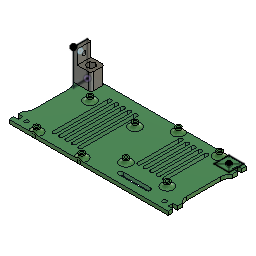
Support_RPI (Autodesk Fusion 360 design; units mm, degrees)
Autodesk Fusion 360 part; units mm, degrees
note: some values were not read from the file. Chosen so that the rebuilt part matches the saved one: that a step has no effect. Set by a fixed rule: which sketch regions a step uses.
sketch "Sketch1" plane through (0, 0, 0) normal (0, 0, 1) x (1, 0, 0) in component "Support_RPI"
  line L0 (-82.5, 42.5) -> (82.5, 42.5)
  line L1 (82.5, 42.5) -> (82.5, -42.5)
  line L2 (82.5, -42.5) -> (-82.5, -42.5)
  line L3 (-82.5, -42.5) -> (-82.5, 42.5)
  line L4 (-82.5, 42.5) -> (82.5, -42.5) construction
  line L5 (82.5, 42.5) -> (-82.5, -42.5) construction
  line L6 (0, 42.5) -> (0, -42.5) construction
  line L7 (-82.5, 42.5) -> (-86.5, 42.5)
  line L8 (-86.5, 42.5) -> (-86.5, 27.5)
  line L9 (-86.5, 27.5) -> (-82.5, 27.5)
  line L10 (-82.5, 27.5) -> (-82.5, 42.5)
  line L11 (-82.5, -42.5) -> (-86.5, -42.5)
  line L12 (-86.5, -42.5) -> (-86.5, -27.5)
  line L13 (-86.5, -27.5) -> (-82.5, -27.5)
  line L14 (-82.5, -27.5) -> (-82.5, -42.5)
  line L15 (82.5, 42.5) -> (86.5, 42.5)
  line L16 (86.5, 42.5) -> (86.5, 27.5)
  line L17 (86.5, 27.5) -> (82.5, 27.5)
  line L18 (82.5, 27.5) -> (82.5, 42.5)
  line L19 (82.5, -42.5) -> (86.5, -42.5)
  line L20 (86.5, -27.5) -> (82.5, -27.5)
  line L21 (82.5, -27.5) -> (82.5, -42.5)
  line L22 (86.5, -42.5) -> (86.5, -27.5)
  line L23 (-82.5, -42.5) -> (-67.5, -42.5)
  line L24 (-67.5, -42.5) -> (-67.5, -27.5)
  line L25 (-67.5, -27.5) -> (-82.5, -27.5)
  line L26 (-82.5, -27.5) -> (-82.5, -42.5)
  line L27 (-82.5, 42.5) -> (-67.5, 42.5)
  line L28 (-67.5, 42.5) -> (-67.5, 27.5)
  line L29 (-67.5, 27.5) -> (-82.5, 27.5)
  line L30 (-82.5, 27.5) -> (-82.5, 42.5)
  line L31 (82.5, 42.5) -> (67.5, 42.5)
  line L32 (67.5, 42.5) -> (67.5, 27.5)
  line L33 (67.5, 27.5) -> (82.5, 27.5)
  line L34 (82.5, 27.5) -> (82.5, 42.5)
  line L35 (82.5, -42.5) -> (67.5, -42.5)
  line L36 (67.5, -27.5) -> (82.5, -27.5)
  line L37 (82.5, -27.5) -> (82.5, -42.5)
  line L38 (67.5, -42.5) -> (67.5, -27.5)
  line L39 (-82.5, 27.5) -> (-67.5, 42.5) construction
  line L40 (-82.5, -42.5) -> (-67.5, -27.5) construction
  circle A0 centre (-75, 35) radius 2.1
  circle A1 centre (-75, -35) radius 2.1
  circle A2 centre (75, 35) radius 2.1
  circle A3 centre (75, -35) radius 2.1
  line L41 (-82.5, 42.5) -> (-86.5, 27.5) construction
  line L42 (-81.5, 32.5) -> (-87.5, 32.5)
  line L43 (-87.5, 32.5) -> (-87.5, 37.5)
  line L44 (-87.5, 37.5) -> (-81.5, 37.5)
  line L45 (-81.5, 37.5) -> (-81.5, 32.5)
  line L46 (-81.5, 32.5) -> (-87.5, 37.5) construction
  line L47 (-87.5, 32.5) -> (-81.5, 37.5) construction
  line L48 (-82.5, -27.5) -> (-86.5, -42.5) construction
  line L49 (-81.5, -37.5) -> (-87.5, -37.5)
  line L50 (-87.5, -37.5) -> (-87.5, -32.5)
  line L51 (-87.5, -32.5) -> (-81.5, -32.5)
  line L52 (-81.5, -32.5) -> (-81.5, -37.5)
  line L53 (-81.5, -37.5) -> (-87.5, -32.5) construction
  line L54 (-87.5, -37.5) -> (-81.5, -32.5) construction
  line L55 (81.5, -37.5) -> (87.5, -37.5)
  line L56 (87.5, -37.5) -> (87.5, -32.5)
  line L57 (87.5, -32.5) -> (81.5, -32.5)
  line L58 (81.5, -32.5) -> (81.5, -37.5)
  line L59 (87.5, 37.5) -> (81.5, 37.5)
  line L60 (81.5, 37.5) -> (81.5, 32.5)
  line L61 (87.5, 32.5) -> (87.5, 37.5)
  line L62 (81.5, 32.5) -> (87.5, 32.5)
  point P0 (-82.5, 35)
  point P1 (-84.5, 35)
  point P2 (-84.5, -35)
  dimension "d1" = 85
  dimension "d2" = 165
  dimension "d167" = 15
  dimension "d168" = 4
  dimension "d169" = 15
  dimension "d170" = 4
  dimension "d187" = 15
  dimension "d188" = 15
  dimension "d189" = 15
  dimension "d190" = 15
  dimension "d201" = 4.2
  dimension "d202" = 4.2
  dimension "d206" = 6
  dimension "d207" = 5
  dimension "d208" = 6
  dimension "d209" = 5
  constraint perpendicular L0 L1
  constraint parallel L1 L3
  constraint horizontal L0
  constraint midpoint L2 L6.end
  constraint midpoint origin L5
  constraint midpoint origin L4
  constraint midpoint origin L6
  constraint horizontal L7
  constraint vertical L8
  constraint horizontal L9
  constraint vertical L10
  constraint horizontal L11
  constraint vertical L12
  constraint horizontal L13
  constraint vertical L14
  constraint symmetric L0.start L6 L0.end
  constraint symmetric L2.end L6 L1.end
  constraint symmetric L6 L7.end L15.end
  constraint symmetric L6 L8.end L16.end
  constraint symmetric L6 L9.end L17.end
  constraint symmetric L6 L11.end L19.end
  constraint symmetric L6 L12.end L20.start
  constraint symmetric L6 L13.end L20.end
  constraint horizontal L23
  constraint vertical L24
  constraint horizontal L25
  constraint vertical L26
  constraint horizontal L27
  constraint vertical L28
  constraint horizontal L29
  constraint vertical L30
  constraint symmetric L6 L23.end L35.end
  constraint symmetric L6 L24.end L36.start
  constraint symmetric L6 L27.end L31.end
  constraint symmetric L6 L28.end L32.end
  constraint midpoint L39 A0.centre
  constraint midpoint L40 A1.centre
  constraint symmetric L6 A0 A2
  constraint symmetric L6 A1 A3
  constraint midpoint L10 P0
  constraint horizontal L42
  constraint perpendicular L42 L43
  constraint parallel L42 L44
  constraint parallel L43 L45
  constraint coincident L46 P1
  constraint coincident L47 P1
  constraint midpoint L41 P1
  constraint horizontal L49
  constraint perpendicular L49 L50
  constraint parallel L49 L51
  constraint parallel L50 L52
  constraint coincident L53 P2
  constraint coincident L54 P2
  constraint midpoint L48 P2
  constraint symmetric L6 L42.start L60.end
  constraint symmetric L6 L42.end L61.start
  constraint symmetric L6 L43.end L59.start
  constraint symmetric L6 L44.end L59.end
  constraint symmetric L6 L49.start L55.start
  constraint symmetric L6 L49.end L55.end
  constraint symmetric L6 L50.end L56.end
  constraint symmetric L6 L51.end L57.end
  measures "d1" distance of L0.end L1.end
  measures "d2" distance of L1.end L2.end
  measures "d121" distance of L0.end
  measures "d122" distance of L0.end
  measures "d128" diameter of L0.end
  measures "d167" distance of L7.end L8.end
  measures "d168" distance of L0.start L7.end
  measures "d169" distance of L11.end L12.end
  measures "d170" distance of L2.end L11.end
  measures "d187" distance of L2.end L23.end
  measures "d188" distance of L2.end L13.end
  measures "d189" distance of L0.start L27.end
  measures "d190" distance of L0.start L9.end
  measures "d201" diameter of A0
  measures "d202" diameter of A1
  measures "d206" distance of L43.end L44.end
  measures "d207" distance of L42.end L43.end
  measures "d208" distance of L50.end L51.end
  measures "d209" distance of L49.end L50.end
  measures "d210" distance of L0.end
extrude "Extrude1" add sketch "Sketch1" along normal blind 4 contours L0 L3 L10 L27 L28 L29 L30 L42 L44 L45 | L3 L7 L8 L10 L30 L44 | L0 L1 L2 L3 L24 L25 L28 L29 L32 L33 L36 L38 | L0 L1 L18 L31 L32 L33 L34 L59 L60 L62 | L3 L8 L9 L10 L30 L42 | L1 L15 L16 L18 L34 L59 | L1 L16 L17 L18 L34 L62 | L2 L3 L14 L23 L24 L25 L26 L49 L51 L52 | L3 L12 L13 L14 L26 L51 | L1 L20 L21 L22 L37 L57 | L1 L2 L21 L35 L36 L37 L38 L55 L57 L58 | L3 L11 L12 L14 L26 L49 | L1 L19 L21 L22 L37 L55 makes body 1 in component "Support_RPI"
sketch "Sketch2" plane through (0, 0, 4) normal (0, 0, 1) x (-1, 0, 0) in component "Support_RPI"
  line L0 (86.5, 42.5) -> (-86.5, 42.5)
  line L1 (-82.5, 27.5) -> (-82.5, -27.5)
  line L2 (-86.5, -42.5) -> (86.5, -42.5)
  circle A0 centre (11, -19) radius 3
  circle A1 centre (11, -19) radius 1.6
  circle A2 centre (60, -19) radius 1.6
  circle A3 centre (60, 39) radius 1.6
  circle A4 centre (60, 39) radius 3
  circle A5 centre (11, 39) radius 1.6
  circle A6 centre (11, 39) radius 3
  line L3 (60, -19) -> (11, -19) construction
  line L4 (11, -19) -> (11, 39) construction
  line L5 (11, 39) -> (60, 39) construction
  line L6 (60, 39) -> (60, -19) construction
  line L7 (60, 10) -> (11, 10) construction
  line L8 (37.5, -30) -> (37.5, 30)
  arc A7 (37.5, 30) -> (33.5, 30) centre (35.5, 30) ccw
  line L9 (33.5, 30) -> (33.5, -30)
  arc A8 (33.5, -30) -> (37.5, -30) centre (35.5, -30) ccw
  line L10 (35.5, -30) -> (35.5, 30) construction
  line L11 (23.5, -30) -> (23.5, 30)
  arc A9 (23.5, 30) -> (19.5, 30) centre (21.5, 30) ccw
  line L12 (19.5, 30) -> (19.5, -30)
  arc A10 (19.5, -30) -> (23.5, -30) centre (21.5, -30) ccw
  line L13 (30.5, -30) -> (30.5, 30)
  arc A11 (30.5, 30) -> (26.5, 30) centre (28.5, 30) ccw
  line L14 (26.5, 30) -> (26.5, -30)
  arc A12 (26.5, -30) -> (30.5, -30) centre (28.5, -30) ccw
  line L15 (44.5, -30) -> (44.5, 30)
  arc A13 (44.5, 30) -> (40.5, 30) centre (42.5, 30) ccw
  line L16 (40.5, 30) -> (40.5, -30)
  arc A14 (40.5, -30) -> (44.5, -30) centre (42.5, -30) ccw
  circle A15 centre (60, -19) radius 3
  line L17 (-82.5, -42.5) -> (-82.5, 42.5) construction
  line L18 (5.5, 42.5) -> (65.5, 42.5) construction
  line L19 (65.5, 42.5) -> (65.5, -42.5) construction
  line L20 (65.5, -42.5) -> (5.5, -42.5) construction
  line L21 (5.5, -42.5) -> (5.5, 42.5) construction
  line L22 (5.5, 42.5) -> (65.5, -42.5) construction
  line L23 (65.5, 42.5) -> (5.5, -42.5) construction
  line L24 (0, 0) -> (35.5, 0) construction
  line L25 (-62.5, 19.5) -> (-17.5, 19.5) construction
  line L26 (-17.5, 19.5) -> (-17.5, -37.5) construction
  line L27 (-17.5, -37.5) -> (-62.5, -37.5) construction
  line L28 (-62.5, -37.5) -> (-62.5, 19.5) construction
  line L29 (-62.5, 19.5) -> (-17.5, -37.5) construction
  line L30 (-17.5, 19.5) -> (-62.5, -37.5) construction
  circle A16 centre (-17.5, -37.5) radius 1.6
  circle A17 centre (-62.5, -37.5) radius 1.6
  circle A18 centre (-17.5, 19.5) radius 1.6
  circle A19 centre (-62.5, 19.5) radius 1.6
  circle A20 centre (-17.5, -37.5) radius 3
  circle A21 centre (-62.5, -37.5) radius 3
  circle A22 centre (-17.5, 19.5) radius 3
  circle A23 centre (-62.5, 19.5) radius 3
  line L31 (51.5, -30) -> (51.5, 30)
  arc A24 (51.5, 30) -> (47.5, 30) centre (49.5, 30) ccw
  line L32 (47.5, 30) -> (47.5, -30)
  arc A25 (47.5, -30) -> (51.5, -30) centre (49.5, -30) ccw
  line L33 (-38, -31.5) -> (-38, 13.5)
  arc A26 (-38, 13.5) -> (-42, 13.5) centre (-40, 13.5) ccw
  line L34 (-42, 13.5) -> (-42, -31.5)
  arc A27 (-42, -31.5) -> (-38, -31.5) centre (-40, -31.5) ccw
  line L35 (-40, -31.5) -> (-40, 13.5) construction
  line L36 (-52, -31.5) -> (-52, 13.5)
  arc A28 (-52, 13.5) -> (-56, 13.5) centre (-54, 13.5) ccw
  line L37 (-56, 13.5) -> (-56, -31.5)
  arc A29 (-56, -31.5) -> (-52, -31.5) centre (-54, -31.5) ccw
  line L38 (-45, -31.5) -> (-45, 13.5)
  arc A30 (-45, 13.5) -> (-49, 13.5) centre (-47, 13.5) ccw
  line L39 (-49, 13.5) -> (-49, -31.5)
  arc A31 (-49, -31.5) -> (-45, -31.5) centre (-47, -31.5) ccw
  line L40 (-31, -31.5) -> (-31, 13.5)
  arc A32 (-31, 13.5) -> (-35, 13.5) centre (-33, 13.5) ccw
  line L41 (-35, 13.5) -> (-35, -31.5)
  arc A33 (-35, -31.5) -> (-31, -31.5) centre (-33, -31.5) ccw
  line L42 (-24, -31.5) -> (-24, 13.5)
  arc A34 (-24, 13.5) -> (-28, 13.5) centre (-26, 13.5) ccw
  line L43 (-28, 13.5) -> (-28, -31.5)
  arc A35 (-28, -31.5) -> (-24, -31.5) centre (-26, -31.5) ccw
  line L44 (-25, 35) -> (-55, 35)
  arc A36 (-55, 35) -> (-55, 30) centre (-55, 32.5) ccw
  line L45 (-55, 30) -> (-25, 30)
  arc A37 (-25, 30) -> (-25, 35) centre (-25, 32.5) ccw
  line L46 (-25, 32.5) -> (-55, 32.5) construction
  line L47 (-40, -9) -> (-40, 32.5) construction
  line L48 (-40, 32.5) -> (-40, 42.5) construction
  circle A38 centre (-75, 35) radius 2.1
  circle A39 centre (75, 35) radius 2.1
  circle A40 centre (75, -35) radius 2.1
  circle A41 centre (-75, -35) radius 2.1
  line L49 (-86.5, 42.5) -> (-86.5, 37.5)
  line L50 (-86.5, 27.5) -> (-82.5, 27.5)
  line L51 (-82.5, -27.5) -> (-86.5, -27.5)
  line L52 (-86.5, -27.5) -> (-86.5, -32.5)
  line L53 (86.5, -42.5) -> (86.5, -37.5)
  line L54 (86.5, -27.5) -> (82.5, -27.5)
  line L55 (82.5, 27.5) -> (86.5, 27.5)
  line L56 (86.5, 27.5) -> (86.5, 32.5)
  line L57 (86.5, -37.5) -> (81.5, -37.5)
  line L58 (81.5, -32.5) -> (86.5, -32.5)
  line L59 (86.5, -32.5) -> (86.5, -27.5)
  line L60 (82.5, -27.5) -> (82.5, 27.5)
  line L61 (81.5, -37.5) -> (81.5, -32.5)
  line L62 (86.5, 32.5) -> (81.5, 32.5)
  line L63 (81.5, 32.5) -> (81.5, 37.5)
  line L64 (81.5, 37.5) -> (86.5, 37.5)
  line L65 (86.5, 37.5) -> (86.5, 42.5)
  line L66 (-86.5, 37.5) -> (-81.5, 37.5)
  line L67 (-81.5, 37.5) -> (-81.5, 32.5)
  line L68 (-81.5, 32.5) -> (-86.5, 32.5)
  line L69 (-86.5, 32.5) -> (-86.5, 27.5)
  line L70 (-86.5, -32.5) -> (-81.5, -32.5)
  line L71 (-81.5, -32.5) -> (-81.5, -37.5)
  line L72 (-81.5, -37.5) -> (-86.5, -37.5)
  line L73 (-86.5, -37.5) -> (-86.5, -42.5)
  line L74 (67.5, -42.5) -> (67.5, 42.5) construction
  line L75 (-67.5, -42.5) -> (-67.5, 42.5) construction
  point P0 (35.5, 10)
  point P1 (35.5, 0)
  point P2 (-40, -9)
  point P3 (-40, -9)
  point P4 (-40, 32.5)
  dimension "d5" = 6
  dimension "d6" = 3.2
  dimension "d8" = 3.2
  dimension "d9" = 6
  dimension "d10" = 3.2
  dimension "d11" = 6
  dimension "d12" = 3.2
  dimension "d16" = 49
  dimension "d17" = 58
  dimension "d65" = 4
  dimension "d68" = 7
  dimension "d69" = 0
  dimension "d128" = 6
  dimension "d131" = 3.5
  dimension "d134" = 15
  dimension "d138" = 60
  dimension "d139" = 85
  dimension "d140" = 57
  dimension "d141" = 45
  dimension "d142" = 5
  dimension "d143" = 3.2
  dimension "d144" = 3.2
  dimension "d145" = 3.2
  dimension "d146" = 3.2
  dimension "d147" = 6
  dimension "d148" = 6
  dimension "d149" = 6
  dimension "d150" = 6
  dimension "d151" = 30
  dimension "d152" = 2
  dimension "d153" = 45
  dimension "d156" = 7
  dimension "d157" = 0
  dimension "d162" = 2.5
  dimension "d163" = 10
  dimension "d164" = 30
  dimension "d226" = 15
  dimension "d227" = 15
  dimension "d228" = 2
  dimension "d229" = 5
  constraint concentric A0 A1
  constraint concentric A3 A4
  constraint concentric A5 A6
  constraint horizontal L3
  constraint vertical L4
  constraint horizontal L5
  constraint vertical L6
  constraint coincident A0.centre A1.centre
  constraint coincident A3.centre A4.centre
  constraint coincident A5.centre A6.centre
  constraint midpoint L6 L7.start
  constraint midpoint L4 L7.end
  constraint tangent L8 A7
  constraint tangent A7 L9
  constraint parallel L8 L9
  constraint tangent L9 A8
  constraint tangent L8 A8
  constraint perpendicular L7 L10
  constraint midpoint L7 P0
  constraint concentric A2 A15
  constraint coincident L6 A2.centre
  constraint coincident A2.centre L3.start
  constraint coincident L2 L17.start
  constraint coincident L0 L17.end
  constraint perpendicular L0 L17
  constraint horizontal L18
  constraint perpendicular L18 L19
  constraint parallel L18 L20
  constraint parallel L19 L21
  constraint coincident L22 P1
  constraint coincident L23 P1
  constraint coincident L10 P1
  constraint coincident L24.start origin
  constraint coincident P1 L24.end
  constraint horizontal L24
  constraint horizontal L25
  constraint perpendicular L25 L26
  constraint parallel L25 L27
  constraint parallel L26 L28
  constraint coincident L29 P3
  constraint coincident L30 P3
  constraint coincident L26.end L27.start
  constraint coincident L27.end L28.start
  constraint coincident L25.end L26.start
  constraint coincident L25.start L28.end
  constraint concentric A16 A20
  constraint concentric A17 A21
  constraint concentric A18 A22
  constraint concentric A19 A23
  constraint coincident L10 P0
  constraint midpoint L10 P1
  constraint tangent L33 A26
  constraint tangent A26 L34
  constraint parallel L33 L34
  constraint tangent L34 A27
  constraint tangent L33 A27
  constraint coincident P3 P2
  constraint midpoint L35 P3
  constraint tangent L44 A36
  constraint tangent A36 L45
  constraint parallel L44 L45
  constraint tangent L45 A37
  constraint tangent L44 A37
  constraint perpendicular L43 L46
  constraint midpoint L46 P4
  constraint coincident P4 L47.end
  constraint vertical L47
  constraint coincident L0 L48.end
  constraint perpendicular L0 L48
  constraint vertical L35
  constraint coincident L2 L74.start
  constraint coincident L0 L74.end
  constraint perpendicular L0 L74
  constraint coincident L2 L75.start
  constraint coincident L0 L75.end
  constraint perpendicular L0 L75
  constraint coincident L1.end L17
  measures "d5" diameter of A0
  measures "d6" diameter of A1
  measures "d8" diameter of A2
  measures "d9" diameter of A4
  measures "d10" diameter of A3
  measures "d11" diameter of A6
  measures "d12" diameter of A5
  measures "d16" distance of A2.centre A0.centre
  measures "d17" distance of A2.centre A3.centre
  measures "d65" diameter of A7
  measures "d128" diameter of A15
  measures "d131" distance of L0 L5
  measures "d134" distance of L1.end L17.start
  measures "d138" distance of L18.start L18.end
  measures "d139" distance of L18.start L20.end
  measures "d140" distance of L25.start L27.end
  measures "d141" distance of L26.end L27.end
  measures "d142" distance of L2 L27.end
  measures "d143" diameter of A16
  measures "d144" diameter of A17
  measures "d145" diameter of A18
  measures "d146" diameter of A19
  measures "d147" diameter of A20
  measures "d148" diameter of A21
  measures "d149" diameter of A22
  measures "d150" diameter of A23
  measures "d151" distance of A8.centre P1
  measures "d152" radius of A27
  measures "d153" distance of A27.centre A26.centre
  measures "d162" radius of A36
  measures "d163" distance of P4 L48.end
  measures "d164" distance of A37.centre A36.centre
  measures "d226" horizontal distance of L54.end L74.start
  measures "d227" distance of L17.start L75.start
  measures "d228" distance of L19.end L74.start
  measures "d229" horizontal distance of L27.end L75.start
extrude "Extrude2" add sketch "Sketch2" along normal blind 5 contours A0 | A4 | A6 | A15 | A20 | A21 | A22 | A23 bodies 1 in component "Support_RPI"
extrude "Extrude8" cut sketch "Sketch2" against normal through all contours L8 A7 L9 A8 | L11 A9 L12 A10 | L13 A11 L14 A12 | L15 A13 L16 A14 | L31 A24 L32 A25 | L33 A26 L34 A27 | L36 A28 L37 A29 | L38 A30 L39 A31 | L40 A32 L41 A33 | L42 A34 L43 A35 | L44 A36 L45 A37 bodies 1 in component "Support_RPI"
extrude "Extrude3" cut sketch "Sketch2" against normal through all contours A1 | A2 | A3 | A5 | A16 | A17 | A18 | A19 bodies 1 in component "Support_RPI"
sketch "Sketch2 (1)" plane through (0, 0, 0) normal (0, 0, -1) x (1, 0, 0) in component "Support_RPI"
  line L0 (-40.5, 30) -> (-40.5, -30)
  arc A0 (-44.5, -30) -> (-40.5, -30) centre (-42.5, -30) ccw
  line L1 (-44.5, -30) -> (-44.5, 30)
  arc A1 (-40.5, 30) -> (-44.5, 30) centre (-42.5, 30) ccw
  line L2 (-26.5, 30) -> (-26.5, -30)
  arc A2 (-30.5, -30) -> (-26.5, -30) centre (-28.5, -30) ccw
  line L3 (-30.5, -30) -> (-30.5, 30)
  arc A3 (-26.5, 30) -> (-30.5, 30) centre (-28.5, 30) ccw
  line L4 (-19.5, 30) -> (-19.5, -30)
  arc A4 (-23.5, -30) -> (-19.5, -30) centre (-21.5, -30) ccw
  line L5 (-23.5, -30) -> (-23.5, 30)
  arc A5 (-19.5, 30) -> (-23.5, 30) centre (-21.5, 30) ccw
  line L6 (-86.5, -42.5) -> (86.5, -42.5)
  line L7 (82.5, -27.5) -> (82.5, 27.5)
  line L8 (86.5, 42.5) -> (-86.5, 42.5)
  line L9 (-82.5, 27.5) -> (-82.5, -27.5)
  circle A6 centre (-60, -19) radius 1.6
  circle A7 centre (-11, -19) radius 1.6
  circle A8 centre (-60, 39) radius 1.6
  circle A9 centre (-11, 39) radius 1.6
  line L10 (-63.4641, 39) -> (-61.7321, 36)
  line L11 (-61.7321, 36) -> (-58.2679, 36)
  line L12 (-58.2679, 36) -> (-56.5359, 39)
  line L13 (-56.5359, 39) -> (-58.2679, 42)
  line L14 (-58.2679, 42) -> (-61.7321, 42)
  line L15 (-61.7321, 42) -> (-63.4641, 39)
  line L16 (-7.5359, 39) -> (-9.2679, 42)
  line L17 (-9.2679, 42) -> (-12.7321, 42)
  line L18 (-12.7321, 42) -> (-14.4641, 39)
  line L19 (-14.4641, 39) -> (-12.7321, 36)
  line L20 (-12.7321, 36) -> (-9.2679, 36)
  line L21 (-9.2679, 36) -> (-7.5359, 39)
  line L22 (-14.4641, -19) -> (-12.7321, -22)
  line L23 (-12.7321, -22) -> (-9.2679, -22)
  line L24 (-9.2679, -22) -> (-7.5359, -19)
  line L25 (-7.5359, -19) -> (-9.2679, -16)
  line L26 (-9.2679, -16) -> (-12.7321, -16)
  line L27 (-12.7321, -16) -> (-14.4641, -19)
  line L28 (-58.2679, -16) -> (-61.7321, -16)
  line L29 (-61.7321, -16) -> (-63.4641, -19)
  line L30 (-63.4641, -19) -> (-61.7321, -22)
  line L31 (-61.7321, -22) -> (-58.2679, -22)
  line L32 (-58.2679, -22) -> (-56.5359, -19)
  line L33 (-56.5359, -19) -> (-58.2679, -16)
  line L34 (-33.5, 30) -> (-33.5, -30)
  arc A10 (-37.5, -30) -> (-33.5, -30) centre (-35.5, -30) ccw
  line L35 (-37.5, -30) -> (-37.5, 30)
  arc A11 (-33.5, 30) -> (-37.5, 30) centre (-35.5, 30) ccw
  circle A12 centre (62.5, -37.5) radius 1.6
  circle A13 centre (17.5, -37.5) radius 1.6
  circle A14 centre (62.5, 19.5) radius 1.6
  circle A15 centre (17.5, 19.5) radius 1.6
  line L36 (42, 13.5) -> (42, -31.5)
  arc A16 (38, -31.5) -> (42, -31.5) centre (40, -31.5) ccw
  line L37 (38, -31.5) -> (38, 13.5)
  arc A17 (42, 13.5) -> (38, 13.5) centre (40, 13.5) ccw
  line L38 (-47.5, 30) -> (-47.5, -30)
  arc A18 (-51.5, -30) -> (-47.5, -30) centre (-49.5, -30) ccw
  line L39 (-51.5, -30) -> (-51.5, 30)
  arc A19 (-47.5, 30) -> (-51.5, 30) centre (-49.5, 30) ccw
  line L40 (35, 13.5) -> (35, -31.5)
  arc A20 (31, -31.5) -> (35, -31.5) centre (33, -31.5) ccw
  line L41 (31, -31.5) -> (31, 13.5)
  arc A21 (35, 13.5) -> (31, 13.5) centre (33, 13.5) ccw
  line L42 (49, 13.5) -> (49, -31.5)
  arc A22 (45, -31.5) -> (49, -31.5) centre (47, -31.5) ccw
  line L43 (45, -31.5) -> (45, 13.5)
  arc A23 (49, 13.5) -> (45, 13.5) centre (47, 13.5) ccw
  line L44 (56, 13.5) -> (56, -31.5)
  arc A24 (52, -31.5) -> (56, -31.5) centre (54, -31.5) ccw
  line L45 (52, -31.5) -> (52, 13.5)
  arc A25 (56, 13.5) -> (52, 13.5) centre (54, 13.5) ccw
  line L46 (28, 13.5) -> (28, -31.5)
  arc A26 (24, -31.5) -> (28, -31.5) centre (26, -31.5) ccw
  line L47 (24, -31.5) -> (24, 13.5)
  arc A27 (28, 13.5) -> (24, 13.5) centre (26, 13.5) ccw
  line L48 (19.2321, 16.5) -> (20.9641, 19.5)
  line L49 (20.9641, 19.5) -> (19.2321, 22.5)
  line L50 (19.2321, 22.5) -> (15.7679, 22.5)
  line L51 (15.7679, 22.5) -> (14.0359, 19.5)
  line L52 (14.0359, 19.5) -> (15.7679, 16.5)
  line L53 (15.7679, 16.5) -> (19.2321, 16.5)
  line L54 (19.2321, -40.5) -> (20.9641, -37.5)
  line L55 (20.9641, -37.5) -> (19.2321, -34.5)
  line L56 (19.2321, -34.5) -> (15.7679, -34.5)
  line L57 (15.7679, -34.5) -> (14.0359, -37.5)
  line L58 (14.0359, -37.5) -> (15.7679, -40.5)
  line L59 (15.7679, -40.5) -> (19.2321, -40.5)
  line L60 (64.2321, -40.5) -> (65.9641, -37.5)
  line L61 (65.9641, -37.5) -> (64.2321, -34.5)
  line L62 (64.2321, -34.5) -> (60.7679, -34.5)
  line L63 (60.7679, -34.5) -> (59.0359, -37.5)
  line L64 (59.0359, -37.5) -> (60.7679, -40.5)
  line L65 (60.7679, -40.5) -> (64.2321, -40.5)
  line L66 (64.2321, 16.5) -> (65.9641, 19.5)
  line L67 (65.9641, 19.5) -> (64.2321, 22.5)
  line L68 (64.2321, 22.5) -> (60.7679, 22.5)
  line L69 (60.7679, 22.5) -> (59.0359, 19.5)
  line L70 (59.0359, 19.5) -> (60.7679, 16.5)
  line L71 (60.7679, 16.5) -> (64.2321, 16.5)
  line L72 (55, 30) -> (25, 30)
  arc A28 (25, 35) -> (25, 30) centre (25, 32.5) ccw
  line L73 (25, 35) -> (55, 35)
  arc A29 (55, 30) -> (55, 35) centre (55, 32.5) ccw
  circle A30 centre (75, 35) radius 2.1
  circle A31 centre (-75, 35) radius 2.1
  circle A32 centre (-75, -35) radius 2.1
  circle A33 centre (75, -35) radius 2.1
  line L74 (86.5, 27.5) -> (86.5, 32.5)
  line L75 (-86.5, 42.5) -> (-86.5, 37.5)
  line L76 (-86.5, 27.5) -> (-82.5, 27.5)
  line L77 (-82.5, -27.5) -> (-86.5, -27.5)
  line L78 (-86.5, -27.5) -> (-86.5, -32.5)
  line L79 (86.5, -42.5) -> (86.5, -37.5)
  line L80 (86.5, -27.5) -> (82.5, -27.5)
  line L81 (82.5, 27.5) -> (86.5, 27.5)
  line L82 (-86.5, -32.5) -> (-81.5, -32.5)
  line L83 (-81.5, -37.5) -> (-86.5, -37.5)
  line L84 (-86.5, -37.5) -> (-86.5, -42.5)
  line L85 (86.5, -37.5) -> (81.5, -37.5)
  line L86 (81.5, -37.5) -> (81.5, -32.5)
  line L87 (81.5, -32.5) -> (86.5, -32.5)
  line L88 (86.5, -32.5) -> (86.5, -27.5)
  line L89 (86.5, 32.5) -> (81.5, 32.5)
  line L90 (81.5, 32.5) -> (81.5, 37.5)
  line L91 (81.5, 37.5) -> (86.5, 37.5)
  line L92 (86.5, 37.5) -> (86.5, 42.5)
  line L93 (-86.5, 37.5) -> (-81.5, 37.5)
  line L94 (-81.5, 37.5) -> (-81.5, 32.5)
  line L95 (-81.5, 32.5) -> (-86.5, 32.5)
  line L96 (-86.5, 32.5) -> (-86.5, 27.5)
  line L97 (-81.5, -32.5) -> (-81.5, -37.5)
  point P0 (-60, 39)
  point P1 (-11, 39)
  point P2 (-11, -19)
  point P3 (-60, -19)
  point P4 (17.5, 19.5)
  point P5 (17.5, -37.5)
  point P6 (62.5, -37.5)
  point P7 (62.5, 19.5)
  dimension "d121" = 6
  dimension "d122" = 6
  dimension "d123" = 6
  dimension "d124" = 6
  dimension "d158" = 6
  dimension "d159" = 6
  dimension "d160" = 6
  dimension "d161" = 6
  constraint coincident P0 A8.centre
  constraint coincident P1 A9.centre
  constraint coincident P2 A7.centre
  constraint coincident P3 A6.centre
  constraint horizontal L28
  constraint horizontal L26
  constraint horizontal L11
  constraint horizontal L20
  constraint coincident P4 A15.centre
  constraint coincident P5 A13.centre
  constraint coincident P6 A12.centre
  constraint coincident P7 A14.centre
  constraint horizontal L53
  constraint horizontal L71
  constraint horizontal L65
  constraint horizontal L59
  measures "d121" distance of L28 L31
  measures "d122" distance of L22 L25
  measures "d123" distance of L16 L19
  measures "d124" distance of L11 L14
  measures "d158" distance of L50 L53
  measures "d159" distance of L68 L71
  measures "d160" distance of L62 L65
  measures "d161" distance of L56 L59
extrude "Extrude4" cut sketch "Sketch2 (1)" against normal blind 3 contours L10 L11 L12 L13 L14 L15 | L16 L17 L18 L19 L20 L21 | L22 L23 L24 L25 L26 L27 | L28 L29 L30 L31 L32 L33 | L48 L49 L50 L51 L52 L53 | L54 L55 L56 L57 L58 L59 | L60 L61 L62 L63 L64 L65 | L66 L67 L68 L69 L70 L71 bodies 1 in component "Support_RPI"
fillet "Fillet2" radius 3.5 8 edges at (20.297, -20.5848, 4) (20.297, 36.4152, 4) (65.297, 36.4152, 4) (65.297, -20.5848, 4) (-57.203, -40.0848, 4) (-57.203, 17.9152, 4) (-8.203, -40.0848, 4) (-8.203, 17.9152, 4) on bodies 1 in component "Support_RPI"
fillet "Fillet11" radius 12 4 edges at (-82.5, 27.5, 2) (-82.5, -27.5, 2) (82.5, 27.5, 2) (82.5, -27.5, 2) on bodies 1 in component "Support_RPI"
sketch "Sketch3" plane through (0, 0, 4) normal (0, 0, 1) x (-1, 0, 0) in component "Support_RPI"
  circle A0 centre (60, -19) radius 6.5
  circle A1 centre (-17.5, 19.5) radius 6.5
  line L0 (-35, -31.5) -> (-35, 13.5)
  arc A2 (-31, 13.5) -> (-35, 13.5) centre (-33, 13.5) ccw
  line L1 (-31, 13.5) -> (-31, -31.5)
  arc A3 (-35, -31.5) -> (-31, -31.5) centre (-33, -31.5) ccw
  line L2 (47.5, -30) -> (47.5, 30)
  arc A4 (51.5, 30) -> (47.5, 30) centre (49.5, 30) ccw
  line L3 (51.5, 30) -> (51.5, -30)
  arc A5 (47.5, -30) -> (51.5, -30) centre (49.5, -30) ccw
  line L4 (40.5, -30) -> (40.5, 30)
  arc A6 (44.5, 30) -> (40.5, 30) centre (42.5, 30) ccw
  line L5 (44.5, 30) -> (44.5, -30)
  arc A7 (40.5, -30) -> (44.5, -30) centre (42.5, -30) ccw
  line L6 (33.5, -30) -> (33.5, 30)
  arc A8 (37.5, 30) -> (33.5, 30) centre (35.5, 30) ccw
  line L7 (37.5, 30) -> (37.5, -30)
  arc A9 (33.5, -30) -> (37.5, -30) centre (35.5, -30) ccw
  line L8 (-42, -31.5) -> (-42, 13.5)
  arc A10 (-38, 13.5) -> (-42, 13.5) centre (-40, 13.5) ccw
  line L9 (-38, 13.5) -> (-38, -31.5)
  arc A11 (-42, -31.5) -> (-38, -31.5) centre (-40, -31.5) ccw
  line L10 (-28, -31.5) -> (-28, 13.5)
  arc A12 (-24, 13.5) -> (-28, 13.5) centre (-26, 13.5) ccw
  line L11 (-24, 13.5) -> (-24, -31.5)
  arc A13 (-28, -31.5) -> (-24, -31.5) centre (-26, -31.5) ccw
  line L12 (-56, -31.5) -> (-56, 13.5)
  arc A14 (-52, 13.5) -> (-56, 13.5) centre (-54, 13.5) ccw
  line L13 (-52, 13.5) -> (-52, -31.5)
  arc A15 (-56, -31.5) -> (-52, -31.5) centre (-54, -31.5) ccw
  line L14 (26.5, -30) -> (26.5, 30)
  arc A16 (30.5, 30) -> (26.5, 30) centre (28.5, 30) ccw
  line L15 (30.5, 30) -> (30.5, -30)
  arc A17 (26.5, -30) -> (30.5, -30) centre (28.5, -30) ccw
  line L16 (19.5, -30) -> (19.5, 30)
  arc A18 (23.5, 30) -> (19.5, 30) centre (21.5, 30) ccw
  line L17 (23.5, 30) -> (23.5, -30)
  arc A19 (19.5, -30) -> (23.5, -30) centre (21.5, -30) ccw
  line L18 (-49, -31.5) -> (-49, 13.5)
  arc A20 (-45, 13.5) -> (-49, 13.5) centre (-47, 13.5) ccw
  line L19 (-45, 13.5) -> (-45, -31.5)
  arc A21 (-49, -31.5) -> (-45, -31.5) centre (-47, -31.5) ccw
  line L20 (-25, 30) -> (-55, 30)
  arc A22 (-55, 35) -> (-55, 30) centre (-55, 32.5) ccw
  line L21 (-55, 35) -> (-25, 35)
  arc A23 (-25, 30) -> (-25, 35) centre (-25, 32.5) ccw
  circle A24 centre (75, -35) radius 2.1
  circle A25 centre (-75, 35) radius 2.1
  circle A26 centre (-75, -35) radius 2.1
  circle A27 centre (75, 35) radius 2.1
  circle A28 centre (-62.5, 19.5) radius 6.5
  arc A29 (5.5228, 42.5) -> (16.4772, 42.5) centre (11, 39) ccw
  line L22 (5.5228, 42.5) -> (-86.5, 42.5)
  line L23 (-86.5, 42.5) -> (-86.5, 37.5)
  line L24 (-86.5, 37.5) -> (-81.5, 37.5)
  line L25 (-81.5, 37.5) -> (-81.5, 32.5)
  line L26 (-81.5, 32.5) -> (-86.5, 32.5)
  line L27 (-86.5, 32.5) -> (-86.5, 27.5)
  arc A30 (-82.5, 18.5557) -> (-86.5, 27.5) centre (-94.5, 18.5557) ccw
  line L28 (-82.5, 18.5557) -> (-82.5, -18.5557)
  arc A31 (-86.5, -27.5) -> (-82.5, -18.5557) centre (-94.5, -18.5557) ccw
  line L29 (-86.5, -27.5) -> (-86.5, -32.5)
  line L30 (-86.5, -32.5) -> (-81.5, -32.5)
  line L31 (-81.5, -32.5) -> (-81.5, -37.5)
  line L32 (-81.5, -37.5) -> (-86.5, -37.5)
  line L33 (-86.5, -37.5) -> (-86.5, -42.5)
  line L34 (-86.5, -42.5) -> (-66.6533, -42.5)
  arc A32 (-58.3467, -42.5) -> (-66.6533, -42.5) centre (-62.5, -37.5) ccw
  line L35 (-58.3467, -42.5) -> (-21.6533, -42.5)
  arc A33 (-13.3467, -42.5) -> (-21.6533, -42.5) centre (-17.5, -37.5) ccw
  line L36 (-13.3467, -42.5) -> (86.5, -42.5)
  line L37 (86.5, -42.5) -> (86.5, -37.5)
  line L38 (86.5, -37.5) -> (81.5, -37.5)
  line L39 (81.5, -37.5) -> (81.5, -32.5)
  line L40 (81.5, -32.5) -> (86.5, -32.5)
  line L41 (86.5, -32.5) -> (86.5, -27.5)
  arc A34 (82.5, -18.5557) -> (86.5, -27.5) centre (94.5, -18.5557) ccw
  line L42 (82.5, -18.5557) -> (82.5, 18.5557)
  arc A35 (86.5, 27.5) -> (82.5, 18.5557) centre (94.5, 18.5557) ccw
  line L43 (86.5, 27.5) -> (86.5, 32.5)
  line L44 (86.5, 32.5) -> (81.5, 32.5)
  line L45 (81.5, 32.5) -> (81.5, 37.5)
  line L46 (81.5, 37.5) -> (86.5, 37.5)
  line L47 (86.5, 37.5) -> (86.5, 42.5)
  line L48 (86.5, 42.5) -> (65.4772, 42.5)
  arc A36 (54.5228, 42.5) -> (65.4772, 42.5) centre (60, 39) ccw
  line L49 (54.5228, 42.5) -> (16.4772, 42.5)
  circle A37 centre (11, -19) radius 6.5
  line L50 (-67, -27) -> (-83, -27)
  line L51 (-83, -27) -> (-83, -43)
  line L52 (-83, -43) -> (-67, -43)
  line L53 (-67, -43) -> (-67, -27)
  line L54 (-67, -27) -> (-83, -43) construction
  line L55 (-83, -27) -> (-67, -43) construction
  point P0 (-75, -35)
  dimension "d230" = 16
  dimension "d231" = 16
  constraint horizontal L50
  constraint perpendicular L50 L51
  constraint parallel L50 L52
  constraint parallel L51 L53
  constraint coincident L54 P0
  constraint coincident L55 P0
  constraint coincident P0 A26.centre
  measures "d230" distance of L51.end L52.end
  measures "d231" distance of L50.end L51.end
extrude "Extrude8'" cut sketch "Sketch3" along normal blind 0.5 contours L30 L31 L32 L34 A32 L50 L51 L53 | A32 L53 bodies 1 in component "Support_RPI"
sketch "Sketch9" plane through (0, 0, 4) normal (0, 0, 1) x (-1, 0, 0)
  circle A0 centre (60, -19) radius 6.5
  circle A1 centre (-17.5, 19.5) radius 6.5
  line L0 (-35, -31.5) -> (-35, 13.5)
  arc A2 (-31, 13.5) -> (-35, 13.5) centre (-33, 13.5) ccw
  line L1 (-31, 13.5) -> (-31, -31.5)
  arc A3 (-35, -31.5) -> (-31, -31.5) centre (-33, -31.5) ccw
  line L2 (47.5, -30) -> (47.5, 30)
  arc A4 (51.5, 30) -> (47.5, 30) centre (49.5, 30) ccw
  line L3 (51.5, 30) -> (51.5, -30)
  arc A5 (47.5, -30) -> (51.5, -30) centre (49.5, -30) ccw
  line L4 (40.5, -30) -> (40.5, 30)
  arc A6 (44.5, 30) -> (40.5, 30) centre (42.5, 30) ccw
  line L5 (44.5, 30) -> (44.5, -30)
  arc A7 (40.5, -30) -> (44.5, -30) centre (42.5, -30) ccw
  line L6 (33.5, -30) -> (33.5, 30)
  arc A8 (37.5, 30) -> (33.5, 30) centre (35.5, 30) ccw
  line L7 (37.5, 30) -> (37.5, -30)
  arc A9 (33.5, -30) -> (37.5, -30) centre (35.5, -30) ccw
  line L8 (-42, -31.5) -> (-42, 13.5)
  arc A10 (-38, 13.5) -> (-42, 13.5) centre (-40, 13.5) ccw
  line L9 (-38, 13.5) -> (-38, -31.5)
  arc A11 (-42, -31.5) -> (-38, -31.5) centre (-40, -31.5) ccw
  line L10 (-28, -31.5) -> (-28, 13.5)
  arc A12 (-24, 13.5) -> (-28, 13.5) centre (-26, 13.5) ccw
  line L11 (-24, 13.5) -> (-24, -31.5)
  arc A13 (-28, -31.5) -> (-24, -31.5) centre (-26, -31.5) ccw
  line L12 (-56, -31.5) -> (-56, 13.5)
  arc A14 (-52, 13.5) -> (-56, 13.5) centre (-54, 13.5) ccw
  line L13 (-52, 13.5) -> (-52, -31.5)
  arc A15 (-56, -31.5) -> (-52, -31.5) centre (-54, -31.5) ccw
  line L14 (26.5, -30) -> (26.5, 30)
  arc A16 (30.5, 30) -> (26.5, 30) centre (28.5, 30) ccw
  line L15 (30.5, 30) -> (30.5, -30)
  arc A17 (26.5, -30) -> (30.5, -30) centre (28.5, -30) ccw
  line L16 (19.5, -30) -> (19.5, 30)
  arc A18 (23.5, 30) -> (19.5, 30) centre (21.5, 30) ccw
  line L17 (23.5, 30) -> (23.5, -30)
  arc A19 (19.5, -30) -> (23.5, -30) centre (21.5, -30) ccw
  line L18 (-49, -31.5) -> (-49, 13.5)
  arc A20 (-45, 13.5) -> (-49, 13.5) centre (-47, 13.5) ccw
  line L19 (-45, 13.5) -> (-45, -31.5)
  arc A21 (-49, -31.5) -> (-45, -31.5) centre (-47, -31.5) ccw
  line L20 (-25, 30) -> (-55, 30)
  arc A22 (-55, 35) -> (-55, 30) centre (-55, 32.5) ccw
  line L21 (-55, 35) -> (-25, 35)
  arc A23 (-25, 30) -> (-25, 35) centre (-25, 32.5) ccw
  circle A24 centre (-75, 35) radius 2.1
  circle A25 centre (-75, -35) radius 2.1
  circle A26 centre (75, 35) radius 2.1
  circle A27 centre (75, -35) radius 2.1
  circle A28 centre (-62.5, 19.5) radius 6.5
  arc A29 (5.5228, 42.5) -> (16.4772, 42.5) centre (11, 39) ccw
  line L22 (86.5, 42.5) -> (65.4772, 42.5)
  line L23 (-86.5, 42.5) -> (-86.5, 37.5)
  line L24 (-86.5, 37.5) -> (-81.5, 37.5)
  line L25 (-81.5, 37.5) -> (-81.5, 32.5)
  line L26 (-81.5, 32.5) -> (-86.5, 32.5)
  arc A30 (-82.5, 18.5557) -> (-86.5, 27.5) centre (-94.5, 18.5557) ccw
  line L27 (-82.5, 18.5557) -> (-82.5, -18.5557)
  arc A31 (-86.5, -27.5) -> (-82.5, -18.5557) centre (-94.5, -18.5557) ccw
  line L28 (-86.5, -37.5) -> (-86.5, -42.5)
  line L29 (-86.5, -32.5) -> (-81.5, -32.5)
  line L30 (-81.5, -32.5) -> (-81.5, -37.5)
  line L31 (-81.5, -37.5) -> (-86.5, -37.5)
  line L32 (-86.5, -42.5) -> (-66.6533, -42.5)
  arc A32 (-67, -42.1904) -> (-66.6533, -42.5) centre (-62.5, -37.5) ccw
  arc A33 (-13.3467, -42.5) -> (-21.6533, -42.5) centre (-17.5, -37.5) ccw
  line L33 (86.5, -42.5) -> (86.5, -37.5)
  line L34 (86.5, -37.5) -> (81.5, -37.5)
  line L35 (81.5, -37.5) -> (81.5, -32.5)
  line L36 (81.5, -32.5) -> (86.5, -32.5)
  arc A34 (82.5, -18.5557) -> (86.5, -27.5) centre (94.5, -18.5557) ccw
  line L37 (82.5, -18.5557) -> (82.5, 18.5557)
  arc A35 (86.5, 27.5) -> (82.5, 18.5557) centre (94.5, 18.5557) ccw
  line L38 (86.5, 27.5) -> (86.5, 32.5)
  line L39 (86.5, 32.5) -> (81.5, 32.5)
  line L40 (81.5, 32.5) -> (81.5, 37.5)
  line L41 (81.5, 37.5) -> (86.5, 37.5)
  arc A36 (54.5228, 42.5) -> (65.4772, 42.5) centre (60, 39) ccw
  circle A37 centre (11, -19) radius 6.5
  line L42 (82.5, -42.5) -> (67.5, -42.5)
  line L43 (67.5, -42.5) -> (67.5, -27.5)
  line L44 (67.5, -27.5) -> (82.5, -27.5)
  line L45 (82.5, -27.5) -> (82.5, -42.5)
  line L46 (82.5, -42.5) -> (67.5, -27.5) construction
  line L47 (67.5, -42.5) -> (82.5, -27.5) construction
  line L48 (82.5, -27.5) -> (86.5, -27.5)
  line L49 (86.5, -27.5) -> (86.5, -42.5)
  line L50 (86.5, -42.5) -> (82.5, -42.5)
  line L51 (82.5, -42.5) -> (82.5, -27.5)
  line L52 (-67, -42.1904) -> (-67, -32.8096)
  arc A38 (-58.3467, -42.5) -> (-67, -32.8096) centre (-62.5, -37.5) ccw
  line L53 (-58.3467, -42.5) -> (-21.6533, -42.5)
  line L54 (-13.3467, -42.5) -> (86.5, -42.5)
  line L55 (86.5, -32.5) -> (86.5, -27.5)
  line L56 (86.5, 37.5) -> (86.5, 42.5)
  line L57 (54.5228, 42.5) -> (16.4772, 42.5)
  line L58 (5.5228, 42.5) -> (-86.5, 42.5)
  line L59 (-86.5, 32.5) -> (-86.5, 27.5)
  line L60 (-86.5, -27.5) -> (-86.5, -32.5)
  point P0 (75, -35)
  dimension "d210" = 15
  dimension "d211" = 15
  constraint horizontal L42
  constraint perpendicular L42 L43
  constraint parallel L42 L44
  constraint parallel L43 L45
  constraint coincident L46 P0
  constraint coincident L47 P0
  constraint coincident P0 A27.centre
  constraint horizontal L48
  constraint vertical L49
  constraint horizontal L50
  constraint vertical L51
  constraint coincident L33.start L49.end
  measures "d210" distance of L43.end L44.end
  measures "d211" distance of L42.end L43.end
extrude "Extrude9" add sketch "Sketch9" along normal blind 18 separate body contours L34 L35 L36 L42 L43 L44 L45 L51 L54 | L34 L35 L36 L45 L51 makes body 2
extrude "Extrude10" add sketch "Sketch9" against normal blind 4 separate body contours L34 L36 L45 L49 L51 | L34 L35 L36 L45 L51 makes body 3
extrude "Extrude11" add sketch "Sketch9" along normal blind 33 contours L36 L45 L48 L49 L51 L55 | L34 L36 L45 L49 L51 | L33 L34 L45 L49 L50 L51 L54 bodies 2 3
sketch "Sketch10" plane through (-82.5, 0, 0) normal (1, 0, 0) x (0, 1, 0)
  line L0 (27.5, 22) -> (42.5, 22)
  line L1 (42.5, 22) -> (42.5, 37)
  line L2 (42.5, 37) -> (27.5, 37)
  line L3 (27.5, 37) -> (27.5, 22)
  line L4 (42.5, 37) -> (27.5, 22) construction
  circle A0 centre (35, 29.5) radius 2.1
  dimension "d218" = 4.2
  constraint coincident L1.end L2.start
  constraint coincident L0.start L3.end
  constraint midpoint L4 A0.centre
  measures "d218" diameter of A0
extrude "Extrude12" cut sketch "Sketch10" against normal through all contours A0 bodies 2
fillet "Fillet3" radius 3 2 edges at (-67.5, 27.5, 13) (-67.5, 42.5, 13) on bodies 2
sketch "Sketch11" plane through (0, 0, 22) normal (0, 0, 1) x (-1, 0, 0)
  arc A0 (67.5, -39.5) -> (70.5, -42.5) centre (70.5, -39.5) ccw
  line L0 (70.5, -42.5) -> (82.5, -42.5)
  line L1 (82.5, -42.5) -> (82.5, -27.5)
  line L2 (82.5, -27.5) -> (70.5, -27.5)
  arc A1 (70.5, -27.5) -> (67.5, -30.5) centre (70.5, -30.5) ccw
  line L3 (67.5, -30.5) -> (67.5, -39.5)
  circle A2 centre (75, -35) radius 2.1
  line L4 (71, -32.6906) -> (71, -37.3094)
  line L5 (71, -37.3094) -> (75, -39.6188)
  line L6 (75, -39.6188) -> (79, -37.3094)
  line L7 (79, -37.3094) -> (79, -32.6906)
  line L8 (79, -32.6906) -> (75, -30.3812)
  line L9 (75, -30.3812) -> (71, -32.6906)
  point P0 (75, -35)
  dimension "d222" = 8
  constraint coincident P0 A2.centre
  constraint vertical L4
  measures "d222" distance of L6 L9
extrude "Extrude13" cut sketch "Sketch11" against normal blind 12 contours L4 L5 L6 L7 L8 L9 bodies 2
sketch "Sketch13" plane through (-86.5, 0, 0) normal (-1, 0, 0) x (0, -1, 0)
  circle A0 centre (-35, 29.5) radius 2.1
  line L0 (-37.5, 4) -> (-37.5, 0)
  line L1 (-37.5, 0) -> (-32.5, 0)
  line L2 (-32.5, 0) -> (-32.5, 4)
  line L3 (-32.5, 4) -> (-27.5, 4)
  line L4 (-27.5, 4) -> (-27.5, 37)
  line L5 (-27.5, 37) -> (-42.5, 37)
  line L6 (-42.5, 37) -> (-42.5, 4)
  line L7 (-42.5, 4) -> (-37.5, 4)
  line L8 (-27.5, 37) -> (-42.5, 37)
  line L9 (-42.5, 37) -> (-42.5, -0.1)
  line L10 (-42.5, -0.1) -> (-27.5, -0.1)
  line L11 (-27.5, -0.1) -> (-27.5, 37)
  circle A1 centre (-35, 29.5) radius 2.1
  line L12 (-42.5, -0.1) -> (-27.5, -0.1)
  line L13 (-27.5, -0.1) -> (-27.5, -1.6)
  line L14 (-27.5, -1.6) -> (-42.5, -1.6)
  line L15 (-42.5, -1.6) -> (-42.5, -0.1)
  point P0 (-42.5, 0)
  dimension "d234" = 0.1
  dimension "d236" = 1.5
  constraint horizontal L8
  constraint vertical L9
  constraint horizontal L10
  constraint vertical L11
  constraint coincident L4.end L5.start
  constraint coincident L9 P0
  constraint concentric A0 A1
  constraint horizontal L12
  constraint vertical L13
  constraint horizontal L14
  constraint vertical L15
  constraint coincident L10.end L11.start
  measures "d234" distance of L9.end P0
  measures "d236" distance of L9.end L14.end
extrude "Extrude14" add sketch "Sketch13" along normal blind 1.5 separate body makes body 4
extrude "Extrude16" add sketch "Sketch13" against normal blind 1.5 contours L10 L12 L13 L14 L15 bodies 4
form "Form1" [no effect]
component "Support_RPI" placed x (1, 0, 0) y (0, 1, 0) z (0, 0, 1) at (0, 0, 0)
hidden bodies 4
equation "d216 = 18 mm + 15 mm"
named bodies: "Support_RPI_part"
